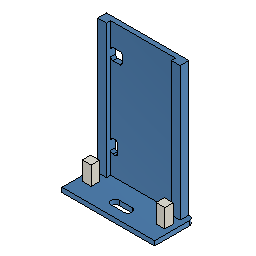
Base Station Enclosure Assembly (Autodesk Fusion 360 archive; units mm, degrees)
design "V2 enclosure Lid"
Autodesk Fusion 360 part; units mm, degrees
sketch "Sketch1" plane through (0, 0, 0) normal (0, 0, 1) x (1, 0, 0)
  line L0 (0, 0) -> (40, 0)
  line L1 (40, 0) -> (40, 17)
  line L2 (40, 17) -> (0, 17)
  line L3 (0, 17) -> (0, 0)
  line L4 (0, 0) -> (0, 6.6)
  line L5 (0, 0) -> (0, 2)
  line L6 (0, 2) -> (40, 2)
  line L7 (0, 17) -> (0, 15)
  line L8 (0, 15) -> (40, 15)
  line L9 (20, 0) -> (20, 4)
  line L10 (20, 4) -> (15.5, 4)
  line L11 (15.5, 4) -> (15.5, 7.5)
  line L12 (20, 4) -> (24.5, 4)
  line L13 (24.5, 4) -> (24.5, 7.5)
  line L14 (15.5, 7.5) -> (24.5, 7.5)
  line L15 (0, 6.6) -> (0, 10.2)
  line L16 (0, 10.2) -> (6, 10.2)
  line L17 (6, 10.2) -> (6, 6.6)
  line L18 (6, 6.6) -> (0, 6.6)
  line L19 (0, 17) -> (2.2, 17)
  line L20 (2.2, 17) -> (2.2, 0)
  line L21 (2.2, 15) -> (6, 15)
  line L22 (6, 15) -> (6, 13.2)
  line L23 (6, 13.2) -> (2.2, 13.2)
  line L24 (34, 6.6) -> (40, 6.6)
  line L25 (34, 10.2) -> (34, 6.6)
  line L26 (40, 10.2) -> (34, 10.2)
  line L27 (34, 13.2) -> (37.8, 13.2)
  line L28 (34, 15) -> (34, 13.2)
  line L29 (37.8, 17) -> (37.8, 0)
  dimension "d1" = 40
  dimension "d2" = 17
  dimension "d3" = 6.6
  dimension "d9" = 2
  dimension "d10" = 2
  dimension "d11" = 4
  dimension "d12" = 4.5
  dimension "d13" = 3.5
  dimension "d14" = 3.6
  dimension "d15" = 6
  dimension "d16" = 2.2
  dimension "d17" = 3.8
  dimension "d18" = 1.8
  constraint horizontal L0
  constraint vertical L1
  constraint horizontal L2
  constraint vertical L3
  constraint coincident L0.start L3.end
  constraint perpendicular L0 L4
  constraint perpendicular L0 L5
  constraint coincident L1 L6.end
  constraint perpendicular L1 L6
  constraint perpendicular L2 L7
  constraint coincident L1 L8.end
  constraint perpendicular L1 L8
  constraint midpoint L0 L9.start
  constraint perpendicular L6 L9
  constraint perpendicular L9 L10
  constraint perpendicular L6 L11
  constraint symmetric L10.start L9 L12.start
  constraint symmetric L9 L10.end L12.end
  constraint symmetric L9 L11.end L13.end
  constraint parallel L3 L15
  constraint perpendicular L3 L16
  constraint perpendicular L16 L17
  constraint perpendicular L4 L18
  constraint perpendicular L3 L19
  constraint coincident L0 L20.end
  constraint perpendicular L0 L20
  constraint coincident L8 L21.start
  constraint coincident L20 L21.start
  constraint perpendicular L20 L21
  constraint perpendicular L21 L22
  constraint coincident L20 L23.end
  constraint perpendicular L20 L23
  constraint symmetric L4.end L9 L24.end
  constraint symmetric L9 L15.end L26.start
  constraint symmetric L9 L16.end L25.start
  constraint symmetric L9 L17.end L24.start
  constraint symmetric L9 L19.end L29.start
  constraint symmetric L9 L20.end L29.end
  constraint symmetric L9 L21.end L28.start
  constraint symmetric L9 L22.end L27.start
  constraint symmetric L9 L23.end L27.end
  measures "d1" distance of L0.start L0.end
  measures "d2" distance of L0.start L2.end
  measures "d3" distance of L0.start L4.end
  measures "d9" distance of L0.start L5.end
  measures "d10" distance of L2.end L7.end
  measures "d11" distance of L9.start L9.end
  measures "d12" distance of L9.end L10.end
  measures "d13" distance of L10.end L11.end
  measures "d14" distance of L4.end L15.end
  measures "d15" distance of L15.end L16.end
  measures "d16" distance of L2.end L19.end
  measures "d17" distance of L21.start L21.end
  measures "d18" distance of L21.end L22.end
extrude "Extrude1" add sketch "Sketch1" along normal blind 2
extrude "Extrude2" add sketch "Sketch1" along normal blind 59.8 contours L2 L8 L20 L21 L29
fillet "Fillet1" [suppressed]
extrude "Extrude3" add sketch "Sketch1" along normal blind 59.8 contours L8 L20 L21 L22 L23 | L8 L27 L28 L29
extrude "Extrude4" add sketch "Sketch1" along normal blind 10 contours L16 L17 L18 L20 | L24 L25 L26 L29
fillet "Fillet2" radius 1.75 4 edges at (24.5, 7.5, 1) (24.5, 4, 1) (15.5, 4, 1) (15.5, 7.5, 1)
sketch "Sketch3" plane through (0, 17, 0) normal (0, 1, 0) x (-1, 0, 0)
  line L0 (0, 2) -> (-2.2, 2)
  line L1 (-2.2, 2) -> (-2.2, 59.8)
  line L2 (-2.2, 59.8) -> (-37.8, 59.8)
  line L3 (-37.8, 59.8) -> (-37.8, 2)
  line L4 (-40, 0) -> (0, 0)
  line L5 (0, 0) -> (0, 2)
  line L6 (-37.8, 2) -> (-40, 2)
  line L7 (-40, 2) -> (-40, 0)
  spline S0 degree 2 poles (-14.8194, 30.1777) (-15.2026, 30.1707) (-15.4828, 30.9322) knots 0 0 0 1 1 1
  spline S1 degree 2 poles (-15.4828, 30.9322) (-15.7629, 31.6937) (-15.7832, 32.8006) knots 0 0 0 1 1 1
  spline S2 degree 2 poles (-15.7832, 32.8006) (-15.8036, 33.9147) (-15.5287, 35.5737) knots 0 0 0 1 1 1
  spline S3 degree 2 poles (-15.5287, 35.5737) (-15.9989, 36.4382) (-16.9027, 37.1457) knots 0 0 0 1 1 1
  spline S4 degree 2 poles (-16.9027, 37.1457) (-17.8065, 37.8531) (-19.4538, 38.6535) knots 0 0 0 1 1 1
  spline S5 degree 2 poles (-19.4538, 38.6535) (-21.1011, 39.4538) (-21.651, 39.8306) knots 0 0 0 1 1 1
  spline S6 degree 2 poles (-21.651, 39.8306) (-22.201, 40.2074) (-22.7242, 40.8722) knots 0 0 0 1 1 1
  spline S7 degree 2 poles (-22.7242, 40.8722) (-24.0767, 42.6291) (-24.1118, 44.545) knots 0 0 0 1 1 1
  spline S8 degree 2 poles (-24.1118, 44.545) (-24.1305, 45.5669) (-23.7096, 46.2241) knots 0 0 0 1 1 1
  spline S9 degree 2 poles (-23.7096, 46.2241) (-23.2886, 46.8813) (-22.6003, 46.8939) knots 0 0 0 1 1 1
  spline S10 degree 2 poles (-22.6003, 46.8939) (-22.2526, 46.9003) (-22.0004, 46.699) knots 0 0 0 1 1 1
  spline S11 degree 2 poles (-22.0004, 46.699) (-21.7483, 46.4978) (-21.7431, 46.214) knots 0 0 0 1 1 1
  spline S12 degree 2 poles (-21.7431, 46.214) (-21.7347, 45.7527) (-22.2172, 45.7439) knots 0 0 0 1 1 1
  spline S13 degree 2 poles (-22.2172, 45.7439) (-22.4443, 45.7397) (-22.6101, 45.8787) knots 0 0 0 1 1 1
  spline S14 degree 2 poles (-22.6101, 45.8787) (-22.7759, 46.0176) (-22.7797, 46.2234) knots 0 0 0 1 1 1
  spline S15 degree 2 poles (-22.7797, 46.2234) (-22.7858, 46.5569) (-22.4594, 46.5629) knots 0 0 0 1 1 1
  spline S16 degree 2 poles (-22.4594, 46.5629) (-22.289, 46.566) (-22.2901, 46.6227) knots 0 0 0 1 1 1
  spline S17 degree 2 poles (-22.2901, 46.6227) (-22.2923, 46.7434) (-22.64, 46.737) knots 0 0 0 1 1 1
  spline S18 degree 2 poles (-22.64, 46.737) (-23.2148, 46.7265) (-23.6013, 46.1267) knots 0 0 0 1 1 1
  spline S19 degree 2 poles (-23.6013, 46.1267) (-23.9878, 45.5269) (-23.972, 44.6612) knots 0 0 0 1 1 1
  spline S20 degree 2 poles (-23.972, 44.6612) (-23.9371, 42.7594) (-22.1922, 41.2794) knots 0 0 0 1 1 1
  spline S21 degree 2 poles (-22.1922, 41.2794) (-21.3774, 40.5845) (-19.5118, 39.4971) knots 0 0 0 1 1 1
  spline S22 degree 2 poles (-19.5118, 39.4971) (-16.4838, 37.7212) (-15.5035, 35.7445) knots 0 0 0 1 1 1
  spline S23 degree 2 poles (-15.5035, 35.7445) (-15.4466, 36.1289) (-15.2904, 36.8984) knots 0 0 0 1 1 1
  spline S24 degree 2 poles (-15.2904, 36.8984) (-14.9331, 38.7079) (-14.9507, 39.6659) knots 0 0 0 1 1 1
  spline S25 degree 2 poles (-14.9507, 39.6659) (-14.9525, 39.7652) (-14.99, 40.2614) knots 0 0 0 1 1 1
  spline S26 degree 2 poles (-14.99, 40.2614) (-15.6083, 39.9165) (-16.4102, 39.9018) knots 0 0 0 1 1 1
  spline S27 degree 2 poles (-16.4102, 39.9018) (-17.9713, 39.8732) (-19.3625, 41.0331) knots 0 0 0 1 1 1
  spline S28 degree 2 poles (-19.3625, 41.0331) (-20.7538, 42.1931) (-20.7785, 43.5413) knots 0 0 0 1 1 1
  spline S29 degree 2 poles (-20.7785, 43.5413) (-20.7887, 44.1019) (-20.4226, 44.46) knots 0 0 0 1 1 1
  spline S30 degree 2 poles (-20.4226, 44.46) (-20.0565, 44.8181) (-19.4675, 44.8289) knots 0 0 0 1 1 1
  spline S31 degree 2 poles (-19.4675, 44.8289) (-18.6586, 44.8437) (-17.6646, 44.2479) knots 0 0 0 1 1 1
  spline S32 degree 2 poles (-17.6646, 44.2479) (-16.6705, 43.6521) (-15.9182, 42.6898) knots 0 0 0 1 1 1
  spline S33 degree 2 poles (-15.9182, 42.6898) (-15.1659, 41.7276) (-14.8536, 40.5691) knots 0 0 0 1 1 1
  spline S34 degree 2 poles (-14.8536, 40.5691) (-14.1046, 41.1432) (-14.1236, 42.1786) knots 0 0 0 1 1 1
  spline S35 degree 2 poles (-14.1236, 42.1786) (-14.1395, 43.0507) (-14.6641, 43.9313) knots 0 0 0 1 1 1
  spline S36 degree 2 poles (-14.6641, 43.9313) (-15.1887, 44.812) (-16.0755, 45.4696) knots 0 0 0 1 1 1
  spline S37 degree 2 poles (-16.0755, 45.4696) (-16.2122, 45.5664) (-16.2129, 45.6019) knots 0 0 0 1 1 1
  spline S38 degree 2 poles (-16.2129, 45.6019) (-16.2137, 45.6444) (-16.1713, 45.6594) knots 0 0 0 1 1 1
  spline S39 degree 2 poles (-16.1713, 45.6594) (-16.0505, 45.6616) (-15.457, 45.0908) knots 0 0 0 1 1 1
  spline S40 degree 2 poles (-15.457, 45.0908) (-14.0382, 43.7194) (-14.0103, 42.1947) knots 0 0 0 1 1 1
  spline S41 degree 2 poles (-14.0103, 42.1947) (-13.9886, 41.0105) (-14.8075, 40.3783) knots 0 0 0 1 1 1
  spline S42 degree 2 poles (-14.8075, 40.3783) (-14.5434, 39.5243) (-14.523, 38.4102) knots 0 0 0 1 1 1
  spline S43 degree 2 poles (-14.523, 38.4102) (-14.5125, 37.8354) (-14.5748, 37.3587) knots 0 0 0 1 1 1
  spline S44 degree 2 poles (-14.5748, 37.3587) (-14.6436, 36.8534) (-15.0121, 34.8804) knots 0 0 0 1 1 1
  spline S45 degree 2 poles (-15.0121, 34.8804) (-14.2653, 33.2543) (-14.2376, 31.7429) knots 0 0 0 1 1 1
  spline S46 degree 2 poles (-14.2376, 31.7429) (-14.2092, 30.1889) (-14.8194, 30.1777) knots 0 0 0 1 1 1
  spline S47 degree 2 poles (-14.8357, 30.291) (-14.6299, 30.2947) (-14.4953, 30.6983) knots 0 0 0 1 1 1
  spline S48 degree 2 poles (-14.4953, 30.6983) (-14.3608, 31.1018) (-14.372, 31.712) knots 0 0 0 1 1 1
  spline S49 degree 2 poles (-14.372, 31.712) (-14.3998, 33.2306) (-15.0645, 34.6452) knots 0 0 0 1 1 1
  spline S50 degree 2 poles (-15.0645, 34.6452) (-15.0897, 34.4673) (-15.2176, 33.6983) knots 0 0 0 1 1 1
  spline S51 degree 2 poles (-15.2176, 33.6983) (-15.4167, 32.5589) (-15.4006, 31.679) knots 0 0 0 1 1 1
  spline S52 degree 2 poles (-15.4006, 31.679) (-15.3901, 31.1042) (-15.2229, 30.6956) knots 0 0 0 1 1 1
  spline S53 degree 2 poles (-15.2229, 30.6956) (-15.0557, 30.2869) (-14.8357, 30.291) knots 0 0 0 1 1 1
  spline S54 degree 2 poles (-16.0675, 40.1849) (-15.4998, 40.1953) (-15.0221, 40.4667) knots 0 0 0 1 1 1
  spline S55 degree 2 poles (-15.0221, 40.4667) (-15.3138, 42.0514) (-16.7155, 43.3957) knots 0 0 0 1 1 1
  spline S56 degree 2 poles (-16.7155, 43.3957) (-18.1172, 44.74) (-19.4513, 44.7156) knots 0 0 0 1 1 1
  spline S57 degree 2 poles (-19.4513, 44.7156) (-19.9622, 44.7062) (-20.3041, 44.3841) knots 0 0 0 1 1 1
  spline S58 degree 2 poles (-20.3041, 44.3841) (-20.646, 44.0619) (-20.6376, 43.6007) knots 0 0 0 1 1 1
  spline S59 degree 2 poles (-20.6376, 43.6007) (-20.6156, 42.4015) (-19.115, 41.279) knots 0 0 0 1 1 1
  spline S60 degree 2 poles (-19.115, 41.279) (-17.6145, 40.1566) (-16.0675, 40.1849) knots 0 0 0 1 1 1
  spline S61 degree 2 poles (-21.3918, 34.5896) (-21.4131, 34.5892) (-21.5784, 34.7141) knots 0 0 0 1 1 1
  line L8 (-21.5784, 34.7141) -> (-21.9665, 35.0124)
  spline S62 degree 2 poles (-21.9665, 35.0124) (-23.8074, 36.4494) (-23.8266, 37.5005) knots 0 0 0 1 1 1
  spline S63 degree 2 poles (-23.8266, 37.5005) (-23.8357, 37.9977) (-23.4835, 38.3416) knots 0 0 0 1 1 1
  spline S64 degree 2 poles (-23.4835, 38.3416) (-23.1314, 38.6855) (-22.5921, 38.6954) knots 0 0 0 1 1 1
  spline S65 degree 2 poles (-22.5921, 38.6954) (-21.3148, 38.7188) (-20.31, 36.9555) knots 0 0 0 1 1 1
  spline S66 degree 2 poles (-20.31, 36.9555) (-19.7819, 36.0282) (-19.7711, 35.4392) knots 0 0 0 1 1 1
  spline S67 degree 2 poles (-19.7711, 35.4392) (-19.7665, 35.1837) (-19.9157, 35) knots 0 0 0 1 1 1
  spline S68 degree 2 poles (-19.9157, 35) (-20.065, 34.8162) (-20.2849, 34.8122) knots 0 0 0 1 1 1
  spline S69 degree 2 poles (-20.2849, 34.8122) (-20.7959, 34.8029) (-21.1664, 35.4633) knots 0 0 0 1 1 1
  spline S70 degree 2 poles (-21.1664, 35.4633) (-21.537, 36.1238) (-21.8778, 37.6792) knots 0 0 0 1 1 1
  spline S71 degree 2 poles (-21.8778, 37.6792) (-22.6175, 38.1483) (-23.1072, 38.1394) knots 0 0 0 1 1 1
  spline S72 degree 2 poles (-23.1072, 38.1394) (-23.7174, 38.1282) (-23.7053, 37.4676) knots 0 0 0 1 1 1
  spline S73 degree 2 poles (-23.7053, 37.4676) (-23.6848, 36.3453) (-21.4657, 34.7587) knots 0 0 0 1 1 1
  spline S74 degree 2 poles (-21.4657, 34.7587) (-21.3508, 34.6757) (-21.3497, 34.6188) knots 0 0 0 1 1 1
  spline S75 degree 2 poles (-21.3497, 34.6188) (-21.3563, 34.5903) (-21.3918, 34.5896) knots 0 0 0 1 1 1
  spline S76 degree 2 poles (-20.0864, 35.2134) (-19.8594, 35.2175) (-19.8639, 35.4659) knots 0 0 0 1 1 1
  spline S77 degree 2 poles (-19.8639, 35.4659) (-19.8708, 35.842) (-20.4036, 36.4462) knots 0 0 0 1 1 1
  spline S78 degree 2 poles (-20.4036, 36.4462) (-20.9364, 37.0505) (-21.7774, 37.6242) knots 0 0 0 1 1 1
  spline S79 degree 2 poles (-21.7774, 37.6242) (-21.4962, 36.6072) (-21.0042, 35.9064) knots 0 0 0 1 1 1
  spline S80 degree 2 poles (-21.0042, 35.9064) (-20.5122, 35.2056) (-20.0864, 35.2134) knots 0 0 0 1 1 1
  spline S81 degree 2 poles (-21.2933, 29.6012) (-21.4425, 29.5985) (-22.6909, 30.6131) knots 0 0 0 1 1 1
  spline S82 degree 2 poles (-22.6909, 30.6131) (-23.7155, 31.433) (-23.7243, 31.9161) knots 0 0 0 1 1 1
  spline S83 degree 2 poles (-23.7243, 31.9161) (-23.7303, 32.2429) (-23.4893, 32.4534) knots 0 0 0 1 1 1
  spline S84 degree 2 poles (-23.4893, 32.4534) (-23.2482, 32.6639) (-22.8792, 32.6707) knots 0 0 0 1 1 1
  spline S85 degree 2 poles (-22.8792, 32.6707) (-22.496, 32.6777) (-22.0448, 32.4588) knots 0 0 0 1 1 1
  spline S86 degree 2 poles (-22.0448, 32.4588) (-23.0513, 33.1502) (-23.4059, 33.5199) knots 0 0 0 1 1 1
  spline S87 degree 2 poles (-23.4059, 33.5199) (-23.7605, 33.8896) (-23.767, 34.2444) knots 0 0 0 1 1 1
  spline S88 degree 2 poles (-23.767, 34.2444) (-23.7739, 34.6205) (-23.4557, 34.8819) knots 0 0 0 1 1 1
  spline S89 degree 2 poles (-23.4557, 34.8819) (-23.1375, 35.1433) (-22.6478, 35.1522) knots 0 0 0 1 1 1
  spline S90 degree 2 poles (-22.6478, 35.1522) (-21.2854, 35.1772) (-20.2, 33.2734) knots 0 0 0 1 1 1
  spline S91 degree 2 poles (-20.2, 33.2734) (-19.7162, 32.4376) (-19.7067, 31.9195) knots 0 0 0 1 1 1
  spline S92 degree 2 poles (-19.7067, 31.9195) (-19.6986, 31.4796) (-20.1244, 31.4718) knots 0 0 0 1 1 1
  spline S93 degree 2 poles (-20.1244, 31.4718) (-20.245, 31.4696) (-20.4447, 31.5227) knots 0 0 0 1 1 1
  line L9 (-20.4447, 31.5227) -> (-19.7498, 31.1734)
  spline S94 degree 2 poles (-19.7498, 31.1734) (-19.7956, 30.9596) (-19.7926, 30.7964) knots 0 0 0 1 1 1
  spline S95 degree 2 poles (-19.7926, 30.7964) (-19.7891, 30.6048) (-19.7338, 30.3006) knots 0 0 0 1 1 1
  line L10 (-19.7338, 30.3006) -> (-21.8359, 31.5185)
  spline S96 degree 2 poles (-21.8359, 31.5185) (-22.9407, 32.1513) (-23.2884, 32.145) knots 0 0 0 1 1 1
  spline S97 degree 2 poles (-23.2884, 32.145) (-23.6219, 32.1389) (-23.6168, 31.8618) knots 0 0 0 1 1 1
  spline S98 degree 2 poles (-23.6168, 31.8618) (-23.6116, 31.5775) (-22.9499, 30.9641) knots 0 0 0 1 1 1
  spline S99 degree 2 poles (-22.9499, 30.9641) (-22.2882, 30.3506) (-21.3239, 29.7215) knots 0 0 0 1 1 1
  spline S100 degree 2 poles (-21.3239, 29.7215) (-21.2521, 29.6801) (-21.2515, 29.6446) knots 0 0 0 1 1 1
  spline S101 degree 2 poles (-21.2515, 29.6446) (-21.2507, 29.602) (-21.2933, 29.6012) knots 0 0 0 1 1 1
  spline S102 degree 2 poles (-20.1547, 31.5777) (-19.807, 31.5841) (-19.8128, 31.9034) knots 0 0 0 1 1 1
  spline S103 degree 2 poles (-19.8128, 31.9034) (-19.8248, 32.5562) (-21.1215, 33.5937) knots 0 0 0 1 1 1
  spline S104 degree 2 poles (-21.1215, 33.5937) (-22.4182, 34.6312) (-23.2059, 34.6167) knots 0 0 0 1 1 1
  spline S105 degree 2 poles (-23.2059, 34.6167) (-23.6672, 34.6083) (-23.6596, 34.1967) knots 0 0 0 1 1 1
  spline S106 degree 2 poles (-23.6596, 34.1967) (-23.6506, 33.7071) (-22.0036, 32.5305) knots 0 0 0 1 1 1
  spline S107 degree 2 poles (-22.0036, 32.5305) (-20.6514, 31.5686) (-20.1547, 31.5777) knots 0 0 0 1 1 1
  spline S108 degree 2 poles (-21.1485, 21.6963) (-21.1699, 21.703) (-21.2635, 21.7651) knots 0 0 0 1 1 1
  line L11 (-21.2635, 21.7651) -> (-21.6884, 22.0629)
  spline S109 degree 2 poles (-21.6884, 22.0629) (-23.5677, 23.3645) (-23.5794, 24.004) knots 0 0 0 1 1 1
  spline S110 degree 2 poles (-23.5794, 24.004) (-23.5855, 24.3379) (-23.341, 24.5556) knots 0 0 0 1 1 1
  spline S111 degree 2 poles (-23.341, 24.5556) (-23.0966, 24.7732) (-22.7063, 24.7804) knots 0 0 0 1 1 1
  spline S112 degree 2 poles (-22.7063, 24.7804) (-22.3089, 24.7877) (-21.8427, 24.5265) knots 0 0 0 1 1 1
  spline S113 degree 2 poles (-21.8427, 24.5265) (-21.7567, 24.4783) (-21.074, 24.0224) knots 0 0 0 1 1 1
  spline S114 degree 2 poles (-21.074, 24.0224) (-20.2115, 23.4419) (-19.949, 23.4467) knots 0 0 0 1 1 1
  spline S115 degree 2 poles (-19.949, 23.4467) (-19.658, 23.452) (-19.6634, 23.743) knots 0 0 0 1 1 1
  spline S116 degree 2 poles (-19.6634, 23.743) (-19.6805, 24.6796) (-23.5683, 26.887) knots 0 0 0 1 1 1
  spline S117 degree 2 poles (-23.5683, 26.887) (-23.5425, 27.0295) (-23.5471, 27.2778) knots 0 0 0 1 1 1
  spline S118 degree 2 poles (-23.5471, 27.2778) (-23.5524, 27.5688) (-23.5846, 27.774) knots 0 0 0 1 1 1
  line L12 (-23.5846, 27.774) -> (-21.9695, 26.7956)
  spline S119 degree 2 poles (-21.9695, 26.7956) (-20.3761, 25.8381) (-20.0213, 25.8446) knots 0 0 0 1 1 1
  spline S120 degree 2 poles (-20.0213, 25.8446) (-19.702, 25.8505) (-19.7068, 26.113) knots 0 0 0 1 1 1
  spline S121 degree 2 poles (-19.7068, 26.113) (-19.7139, 26.5033) (-20.8514, 27.3698) knots 0 0 0 1 1 1
  spline S122 degree 2 poles (-20.8514, 27.3698) (-21.9888, 28.2363) (-23.6085, 29.0797) knots 0 0 0 1 1 1
  spline S123 degree 2 poles (-23.6085, 29.0797) (-23.5831, 29.2434) (-23.5878, 29.4989) knots 0 0 0 1 1 1
  spline S124 degree 2 poles (-23.5878, 29.4989) (-23.5928, 29.7756) (-23.625, 29.9809) knots 0 0 0 1 1 1
  line L13 (-23.625, 29.9809) -> (-22.0098, 28.9954)
  spline S125 degree 2 poles (-22.0098, 28.9954) (-20.3443, 27.9753) (-19.954, 27.9825) knots 0 0 0 1 1 1
  spline S126 degree 2 poles (-19.954, 27.9825) (-19.7411, 27.9864) (-19.7441, 28.1499) knots 0 0 0 1 1 1
  spline S127 degree 2 poles (-19.7441, 28.1499) (-19.7505, 28.4984) (-21.2927, 29.5655) knots 0 0 0 1 1 1
  spline S128 degree 2 poles (-21.2927, 29.5655) (-21.3933, 29.6348) (-21.3941, 29.6775) knots 0 0 0 1 1 1
  spline S129 degree 2 poles (-21.3941, 29.6775) (-21.3875, 29.706) (-21.352, 29.7066) knots 0 0 0 1 1 1
  spline S130 degree 2 poles (-21.352, 29.7066) (-21.2883, 29.7078) (-20.4549, 29.069) knots 0 0 0 1 1 1
  spline S131 degree 2 poles (-20.4549, 29.069) (-19.643, 28.4439) (-19.6366, 28.0957) knots 0 0 0 1 1 1
  spline S132 degree 2 poles (-19.6366, 28.0957) (-19.6325, 27.8683) (-19.8459, 27.7008) knots 0 0 0 1 1 1
  spline S133 degree 2 poles (-19.8459, 27.7008) (-20.0593, 27.5334) (-20.3574, 27.5279) knots 0 0 0 1 1 1
  spline S134 degree 2 poles (-20.3574, 27.5279) (-20.7689, 27.5204) (-21.5075, 27.9256) knots 0 0 0 1 1 1
  spline S135 degree 2 poles (-21.5075, 27.9256) (-19.6107, 26.6827) (-19.5993, 26.0582) knots 0 0 0 1 1 1
  spline S136 degree 2 poles (-19.5993, 26.0582) (-19.5938, 25.7602) (-19.8316, 25.5642) knots 0 0 0 1 1 1
  spline S137 degree 2 poles (-19.8316, 25.5642) (-20.0694, 25.3682) (-20.4313, 25.3615) knots 0 0 0 1 1 1
  spline S138 degree 2 poles (-20.4313, 25.3615) (-20.8357, 25.3541) (-21.4671, 25.7188) knots 0 0 0 1 1 1
  spline S139 degree 2 poles (-21.4671, 25.7188) (-19.569, 24.4048) (-19.5567, 23.7307) knots 0 0 0 1 1 1
  spline S140 degree 2 poles (-19.5567, 23.7307) (-19.5511, 23.4256) (-19.8098, 23.2114) knots 0 0 0 1 1 1
  spline S141 degree 2 poles (-19.8098, 23.2114) (-20.0685, 22.9973) (-20.4446, 22.9904) knots 0 0 0 1 1 1
  spline S142 degree 2 poles (-20.4446, 22.9904) (-20.8846, 22.9824) (-21.4799, 23.3193) knots 0 0 0 1 1 1
  spline S143 degree 2 poles (-21.4799, 23.3193) (-21.4871, 23.3262) (-22.3994, 23.9129) knots 0 0 0 1 1 1
  spline S144 degree 2 poles (-22.3994, 23.9129) (-22.9167, 24.2512) (-23.1863, 24.2463) knots 0 0 0 1 1 1
  spline S145 degree 2 poles (-23.1863, 24.2463) (-23.4772, 24.241) (-23.4719, 23.9496) knots 0 0 0 1 1 1
  spline S146 degree 2 poles (-23.4719, 23.9496) (-23.4618, 23.3953) (-21.6473, 22.1491) knots 0 0 0 1 1 1
  line L14 (-21.6473, 22.1491) -> (-21.3377, 21.9345)
  line L15 (-21.3377, 21.9345) -> (-21.179, 21.8094)
  spline S147 degree 2 poles (-21.179, 21.8094) (-21.1073, 21.7751) (-21.1067, 21.7396) knots 0 0 0 1 1 1
  spline S148 degree 2 poles (-21.1067, 21.7396) (-21.1059, 21.697) (-21.1485, 21.6963) knots 0 0 0 1 1 1
  spline S149 degree 2 poles (-17.6126, 13.8995) (-19.2386, 13.8697) (-21.1073, 15.4599) knots 0 0 0 1 1 1
  spline S150 degree 2 poles (-21.1073, 15.4599) (-23.3803, 17.3974) (-23.4111, 19.0781) knots 0 0 0 1 1 1
  spline S151 degree 2 poles (-23.4111, 19.0781) (-23.4267, 19.9312) (-22.8289, 20.4861) knots 0 0 0 1 1 1
  spline S152 degree 2 poles (-22.8289, 20.4861) (-22.2312, 21.0411) (-21.2788, 21.0586) knots 0 0 0 1 1 1
  spline S153 degree 2 poles (-21.2788, 21.0586) (-19.3712, 21.0935) (-17.3568, 18.7865) knots 0 0 0 1 1 1
  spline S154 degree 2 poles (-17.3568, 18.7865) (-15.6248, 16.7938) (-15.6027, 15.5867) knots 0 0 0 1 1 1
  spline S155 degree 2 poles (-15.6027, 15.5867) (-15.589, 14.8362) (-16.1403, 14.3763) knots 0 0 0 1 1 1
  spline S156 degree 2 poles (-16.1403, 14.3763) (-16.6917, 13.9164) (-17.6126, 13.8995) knots 0 0 0 1 1 1
  spline S157 degree 2 poles (-16.8415, 14.4318) (-15.6813, 14.4531) (-15.7018, 15.5707) knots 0 0 0 1 1 1
  spline S158 degree 2 poles (-15.7018, 15.5707) (-15.7186, 16.4868) (-16.8185, 17.6671) knots 0 0 0 1 1 1
  spline S159 degree 2 poles (-16.8185, 17.6671) (-17.8607, 18.7917) (-19.3154, 19.5819) knots 0 0 0 1 1 1
  spline S160 degree 2 poles (-19.3154, 19.5819) (-20.8416, 20.4064) (-21.9976, 20.3852) knots 0 0 0 1 1 1
  spline S161 degree 2 poles (-21.9976, 20.3852) (-23.3352, 20.3607) (-23.312, 19.0941) knots 0 0 0 1 1 1
  spline S162 degree 2 poles (-23.312, 19.0941) (-23.2834, 17.5341) (-21.0749, 15.9999) knots 0 0 0 1 1 1
  spline S163 degree 2 poles (-21.0749, 15.9999) (-20.0317, 15.2742) (-18.8733, 14.845) knots 0 0 0 1 1 1
  spline S164 degree 2 poles (-18.8733, 14.845) (-17.7148, 14.4158) (-16.8415, 14.4318) knots 0 0 0 1 1 1
  spline S165 degree 2 poles (-16.7428, 7.3707) (-18.4229, 7.3399) (-18.9868, 10.2542) knots 0 0 0 1 1 1
  spline S166 degree 2 poles (-18.9868, 10.2542) (-19.346, 8.5298) (-20.7024, 8.5049) knots 0 0 0 1 1 1
  spline S167 degree 2 poles (-20.7024, 8.5049) (-21.7252, 8.4862) (-22.5207, 9.6418) knots 0 0 0 1 1 1
  spline S168 degree 2 poles (-22.5207, 9.6418) (-23.3162, 10.7974) (-23.3443, 12.3358) knots 0 0 0 1 1 1
  spline S169 degree 2 poles (-23.3443, 12.3358) (-23.3622, 13.3095) (-22.9834, 13.9421) knots 0 0 0 1 1 1
  spline S170 degree 2 poles (-22.9834, 13.9421) (-22.6045, 14.5747) (-21.9943, 14.5859) knots 0 0 0 1 1 1
  spline S171 degree 2 poles (-21.9943, 14.5859) (-21.3627, 14.5975) (-20.9043, 13.9847) knots 0 0 0 1 1 1
  spline S172 degree 2 poles (-20.9043, 13.9847) (-20.4459, 13.372) (-20.4298, 12.4921) knots 0 0 0 1 1 1
  spline S173 degree 2 poles (-20.4298, 12.4921) (-20.4175, 11.8251) (-20.5027, 11.8235) knots 0 0 0 1 1 1
  spline S174 degree 2 poles (-20.5027, 11.8235) (-20.5453, 11.8228) (-20.546, 11.8653) knots 0 0 0 1 1 1
  line L16 (-20.546, 11.8653) -> (-20.5471, 11.9221)
  spline S175 degree 2 poles (-20.5471, 11.9221) (-20.5093, 12.1854) (-20.5126, 12.3628) knots 0 0 0 1 1 1
  spline S176 degree 2 poles (-20.5126, 12.3628) (-20.5267, 13.1363) (-20.9801, 13.6639) knots 0 0 0 1 1 1
  spline S177 degree 2 poles (-20.9801, 13.6639) (-21.4334, 14.1916) (-22.072, 14.1799) knots 0 0 0 1 1 1
  spline S178 degree 2 poles (-22.072, 14.1799) (-22.5971, 14.1702) (-22.9229, 13.7409) knots 0 0 0 1 1 1
  spline S179 degree 2 poles (-22.9229, 13.7409) (-23.2486, 13.3116) (-23.2364, 12.643) knots 0 0 0 1 1 1
  spline S180 degree 2 poles (-23.2364, 12.643) (-23.2126, 11.3458) (-22.2694, 10.2745) knots 0 0 0 1 1 1
  spline S181 degree 2 poles (-22.2694, 10.2745) (-21.3261, 9.2033) (-20.2183, 9.2236) knots 0 0 0 1 1 1
  spline S182 degree 2 poles (-20.2183, 9.2236) (-19.3021, 9.2404) (-19.0315, 10.3669) knots 0 0 0 1 1 1
  spline S183 degree 2 poles (-19.0315, 10.3669) (-19.1349, 10.9755) (-19.1421, 11.3658) knots 0 0 0 1 1 1
  spline S184 degree 2 poles (-19.1421, 11.3658) (-19.1488, 11.7348) (-19.0566, 11.7364) knots 0 0 0 1 1 1
  spline S185 degree 2 poles (-19.0566, 11.7364) (-18.9146, 11.739) (-18.905, 11.2139) knots 0 0 0 1 1 1
  spline S186 degree 2 poles (-18.905, 11.2139) (-18.8976, 10.8095) (-18.9605, 10.3682) knots 0 0 0 1 1 1
  spline S187 degree 2 poles (-18.9605, 10.3682) (-18.5792, 9.2962) (-17.887, 8.6701) knots 0 0 0 1 1 1
  spline S188 degree 2 poles (-17.887, 8.6701) (-17.1948, 8.0439) (-16.3937, 8.0585) knots 0 0 0 1 1 1
  spline S189 degree 2 poles (-16.3937, 8.0585) (-15.4935, 8.075) (-15.5146, 9.2246) knots 0 0 0 1 1 1
  spline S190 degree 2 poles (-15.5146, 9.2246) (-15.5328, 10.218) (-16.234, 11.199) knots 0 0 0 1 1 1
  spline S191 degree 2 poles (-16.234, 11.199) (-16.9352, 12.1799) (-17.6287, 12.1672) knots 0 0 0 1 1 1
  spline S192 degree 2 poles (-17.6287, 12.1672) (-18.2657, 12.1555) (-18.2507, 11.3359) knots 0 0 0 1 1 1
  spline S193 degree 2 poles (-18.2507, 11.3359) (-18.2417, 10.8471) (-17.8386, 10.2379) knots 0 0 0 1 1 1
  spline S194 degree 2 poles (-17.8386, 10.2379) (-17.4355, 9.6287) (-16.8924, 9.2844) knots 0 0 0 1 1 1
  spline S195 degree 2 poles (-16.8924, 9.2844) (-16.8212, 9.2502) (-16.8203, 9.2007) knots 0 0 0 1 1 1
  spline S196 degree 2 poles (-16.8203, 9.2007) (-16.8268, 9.1722) (-16.848, 9.1718) knots 0 0 0 1 1 1
  spline S197 degree 2 poles (-16.848, 9.1718) (-16.9256, 9.1704) (-17.2272, 9.4341) knots 0 0 0 1 1 1
  spline S198 degree 2 poles (-17.2272, 9.4341) (-17.5288, 9.6979) (-17.7167, 9.9284) knots 0 0 0 1 1 1
  spline S199 degree 2 poles (-17.7167, 9.9284) (-18.3236, 10.6685) (-18.3363, 11.3628) knots 0 0 0 1 1 1
  spline S200 degree 2 poles (-18.3363, 11.3628) (-18.344, 11.783) (-18.1047, 12.051) knots 0 0 0 1 1 1
  spline S201 degree 2 poles (-18.1047, 12.051) (-17.8653, 12.319) (-17.483, 12.326) knots 0 0 0 1 1 1
  spline S202 degree 2 poles (-17.483, 12.326) (-16.7681, 12.3391) (-16.109, 11.3432) knots 0 0 0 1 1 1
  spline S203 degree 2 poles (-16.109, 11.3432) (-15.45, 10.3473) (-15.4292, 9.212) knots 0 0 0 1 1 1
  spline S204 degree 2 poles (-15.4292, 9.212) (-15.414, 8.3817) (-15.77, 7.8819) knots 0 0 0 1 1 1
  spline S205 degree 2 poles (-15.77, 7.8819) (-16.126, 7.382) (-16.7428, 7.3707) knots 0 0 0 1 1 1
sketch "Sketch4" plane through (0, 17, 0) normal (0, 1, 0) x (-1, 0, 0)
  line L0 (-40, 0) -> (0, 0)
  line L1 (0, 0) -> (0, 2)
  line L2 (0, 2) -> (-2.2, 2)
  line L3 (-2.2, 2) -> (-2.2, 59.8)
  line L4 (-2.2, 59.8) -> (-37.8, 59.8)
  line L5 (-37.8, 59.8) -> (-37.8, 2)
  line L6 (-37.8, 2) -> (-40, 2)
  line L7 (-40, 2) -> (-40, 0)
  line L8 (-35.4636, 42.0484) -> (-35.4636, 17.9538) construction
  line L9 (-35.4636, 17.9538) -> (-7.8615, 17.9538) construction
  line L10 (-7.8615, 17.9538) -> (-7.8615, 42.0484) construction
  line L11 (-7.8615, 42.0484) -> (-35.4636, 42.0484) construction
  dimension "d45" = 6
  text T0 "TEAM\n03" font "Arial Black" height 6 align centre middle in box 24.0946 x 27.6021 at (-35.4636, 42.0484) x (0, -1) y (1, 0) spacing 1 kerned
extrude "Extrude8" cut sketch "Sketch4" against normal blind 1 text T0
sketch "Sketch5" plane through (0, 17, 0) normal (0, 1, 0) x (-1, 0, 0)
  line L0 (-18.7526, 31.3599) -> (-18.7526, 36.4185)
  line L1 (-18.7526, 36.4185) -> (-12.7526, 36.4185)
  line L2 (-12.7526, 36.4185) -> (-12.7526, 31.4499)
  line L3 (-12.7526, 31.4499) -> (-14.0336, 31.4499)
  line L4 (-14.0336, 31.4499) -> (-14.0336, 34.5604)
  line L5 (-14.0336, 34.5604) -> (-14.9873, 34.5604)
  line L6 (-14.9873, 34.5604) -> (-14.9873, 31.675)
  line L7 (-14.9873, 31.675) -> (-16.211, 31.675)
  line L8 (-16.211, 31.675) -> (-16.211, 34.5604)
  line L9 (-16.211, 34.5604) -> (-17.3938, 34.5604)
  line L10 (-17.3938, 34.5604) -> (-17.3938, 31.3599)
  line L11 (-17.3938, 31.3599) -> (-18.7526, 31.3599)
  spline S0 degree 3 poles (-25.5057, 27.1239) (-25.5119, 27.2162) (-25.5238, 27.3939) (-25.6318, 27.5349) (-25.6837, 27.6027) knots 0 0 0 0 0.027074 0.052111 0.052111 0.052111 0.052111
  spline S1 degree 3 poles (-25.6837, 27.6027) (-25.7629, 27.6602) (-25.9488, 27.7952) (-26.1769, 27.8315) (-26.3079, 27.8524) knots 0 0 0 0 0.028969 0.068055 0.068055 0.068055 0.068055
  line L12 (-26.3079, 27.8524) -> (-26.0255, 29.4281)
  spline S2 degree 3 poles (-26.0255, 29.4281) (-25.7916, 29.3509) (-25.339, 29.2014) (-25.0237, 28.8451) (-24.8713, 28.673) knots 0 0 0 0 0.072436 0.140136 0.140136 0.140136 0.140136
  spline S3 degree 3 poles (-24.8713, 28.673) (-24.7547, 28.4525) (-24.4939, 27.9596) (-24.4786, 27.4003) (-24.4702, 27.0911) knots 0 0 0 0 0.073881 0.16514 0.16514 0.16514 0.16514
  spline S4 degree 3 poles (-24.4702, 27.0911) (-24.4753, 26.7449) (-24.4841, 26.1397) (-24.7811, 25.6165) (-24.9081, 25.3926) knots 0 0 0 0 0.101784 0.177892 0.177892 0.177892 0.177892
  spline S5 degree 3 poles (-24.9081, 25.3926) (-25.0625, 25.2398) (-25.3687, 24.9368) (-25.7969, 24.8913) (-26.0091, 24.8688) knots 0 0 0 0 0.063135 0.125208 0.125208 0.125208 0.125208
  spline S6 degree 3 poles (-26.0091, 24.8688) (-26.1353, 24.8774) (-26.3863, 24.8946) (-26.6046, 25.0195) (-26.713, 25.0816) knots 0 0 0 0 0.03742 0.074398 0.074398 0.074398 0.074398
  spline S7 degree 3 poles (-26.713, 25.0816) (-26.8171, 25.1658) (-27.04, 25.3461) (-27.1871, 25.5927) (-27.2656, 25.7241) knots 0 0 0 0 0.039844 0.085338 0.085338 0.085338 0.085338
  spline S8 degree 3 poles (-27.2656, 25.7241) (-27.2924, 25.6202) (-27.34, 25.4354) (-27.4278, 25.2661) (-27.4661, 25.1921) knots 0 0 0 0 0.032077 0.05702 0.05702 0.05702 0.05702
  spline S9 degree 3 poles (-27.4661, 25.1921) (-27.5321, 25.0982) (-27.6633, 24.9115) (-27.8555, 24.7886) (-27.9511, 24.7276) knots 0 0 0 0 0.034061 0.067736 0.067736 0.067736 0.067736
  spline S10 degree 3 poles (-27.9511, 24.7276) (-28.0595, 24.6792) (-28.2878, 24.5774) (-28.538, 24.5672) (-28.6694, 24.5618) knots 0 0 0 0 0.035262 0.074313 0.074313 0.074313 0.074313
  spline S11 degree 3 poles (-28.6694, 24.5618) (-28.8434, 24.5739) (-29.1964, 24.5984) (-29.5134, 24.756) (-29.6742, 24.836) knots 0 0 0 0 0.051769 0.105062 0.105062 0.105062 0.105062
  spline S12 degree 3 poles (-29.6742, 24.836) (-29.8257, 24.9384) (-30.1323, 25.1456) (-30.32, 25.4646) (-30.415, 25.6259) knots 0 0 0 0 0.054141 0.109515 0.109515 0.109515 0.109515
  spline S13 degree 3 poles (-30.415, 25.6259) (-30.4906, 25.8226) (-30.6579, 26.2577) (-30.6688, 26.7247) (-30.6749, 26.9806) knots 0 0 0 0 0.062756 0.138852 0.138852 0.138852 0.138852
  spline S14 degree 3 poles (-30.6749, 26.9806) (-30.6714, 27.2267) (-30.6653, 27.6664) (-30.5384, 28.0868) (-30.4825, 28.2719) knots 0 0 0 0 0.073367 0.131116 0.131116 0.131116 0.131116
  spline S15 degree 3 poles (-30.4825, 28.2719) (-30.412, 28.4216) (-30.2732, 28.7163) (-30.0363, 28.9397) (-29.9197, 29.0495) knots 0 0 0 0 0.049159 0.096753 0.096753 0.096753 0.096753
  spline S16 degree 3 poles (-29.9197, 29.0495) (-29.784, 29.1465) (-29.4982, 29.3508) (-29.1641, 29.4605) (-28.9886, 29.5181) knots 0 0 0 0 0.049739 0.104776 0.104776 0.104776 0.104776
  line L13 (-28.9886, 29.5181) -> (-28.7676, 27.8524)
  spline S17 degree 3 poles (-28.7676, 27.8524) (-28.915, 27.8221) (-29.1705, 27.7696) (-29.3778, 27.6135) (-29.4654, 27.5475) knots 0 0 0 0 0.044421 0.076985 0.076985 0.076985 0.076985
  spline S18 degree 3 poles (-29.4654, 27.5475) (-29.5221, 27.4722) (-29.6393, 27.3167) (-29.6529, 27.1221) (-29.6598, 27.0215) knots 0 0 0 0 0.027641 0.057153 0.057153 0.057153 0.057153
  spline S19 degree 3 poles (-29.6598, 27.0215) (-29.6497, 26.9145) (-29.6296, 26.7011) (-29.4859, 26.5421) (-29.4143, 26.4629) knots 0 0 0 0 0.031354 0.062502 0.062502 0.062502 0.062502
  spline S20 degree 3 poles (-29.4143, 26.4629) (-29.322, 26.3979) (-29.1262, 26.2599) (-28.8863, 26.2468) (-28.7594, 26.2398) knots 0 0 0 0 0.033176 0.070431 0.070431 0.070431 0.070431
  spline S21 degree 3 poles (-28.7594, 26.2398) (-28.6317, 26.2456) (-28.3949, 26.2563) (-28.2018, 26.3921) (-28.1128, 26.4547) knots 0 0 0 0 0.037427 0.06941 0.06941 0.06941 0.06941
  spline S22 degree 3 poles (-28.1128, 26.4547) (-28.046, 26.5353) (-27.906, 26.704) (-27.8913, 26.9233) (-27.8836, 27.0379) knots 0 0 0 0 0.030607 0.064099 0.064099 0.064099 0.064099
  spline S23 degree 3 poles (-27.8836, 27.0379) (-27.8896, 27.1161) (-27.9038, 27.2993) (-27.9534, 27.4765) (-27.9818, 27.5782) knots 0 0 0 0 0.023458 0.055025 0.055025 0.055025 0.055025
  line L14 (-27.9818, 27.5782) -> (-26.7908, 27.4922)
  spline S24 degree 3 poles (-26.7908, 27.4922) (-26.7967, 27.451) (-26.8071, 27.379) (-26.81, 27.3064) (-26.8113, 27.2753) knots 0 0 0 0 0.012475 0.021801 0.021801 0.021801 0.021801
  spline S25 degree 3 poles (-26.8113, 27.2753) (-26.8034, 27.1715) (-26.7879, 26.9685) (-26.6634, 26.8076) (-26.6025, 26.7289) knots 0 0 0 0 0.030481 0.059646 0.059646 0.059646 0.059646
  spline S26 degree 3 poles (-26.6025, 26.7289) (-26.5305, 26.6651) (-26.3885, 26.5393) (-26.2001, 26.5196) (-26.1073, 26.51) knots 0 0 0 0 0.028112 0.055373 0.055373 0.055373 0.055373
  spline S27 degree 3 poles (-26.1073, 26.51) (-26.022, 26.5154) (-25.859, 26.5258) (-25.7306, 26.6259) (-25.6694, 26.6737) knots 0 0 0 0 0.024996 0.047731 0.047731 0.047731 0.047731
  spline S28 degree 3 poles (-25.6694, 26.6737) (-25.6217, 26.7359) (-25.5202, 26.8683) (-25.5107, 27.0354) (-25.5057, 27.1239) knots 0 0 0 0 0.022993 0.048899 0.048899 0.048899 0.048899
  spline S29 degree 3 poles (-29.7253, 34.6014) (-29.5967, 34.6712) (-29.3108, 34.8265) (-28.9934, 34.8991) (-28.8188, 34.939) knots 0 0 0 0 0.043723 0.097138 0.097138 0.097138 0.097138
  spline S30 degree 3 poles (-28.8188, 34.939) (-28.6175, 34.9742) (-28.1972, 35.0477) (-27.7704, 35.0556) (-27.548, 35.0597) knots 0 0 0 0 0.061196 0.127823 0.127823 0.127823 0.127823
  spline S31 degree 3 poles (-27.548, 35.0597) (-27.0496, 35.0561) (-26.194, 35.0497) (-25.4601, 34.6222) (-25.1537, 34.4438) knots 0 0 0 0 0.146209 0.250976 0.250976 0.250976 0.250976
  spline S32 degree 3 poles (-25.1537, 34.4438) (-24.9548, 34.1956) (-24.5181, 33.6508) (-24.4871, 32.9492) (-24.4702, 32.5673) knots 0 0 0 0 0.093096 0.204358 0.204358 0.204358 0.204358
  spline S33 degree 3 poles (-24.4702, 32.5673) (-24.4737, 32.382) (-24.4801, 32.0436) (-24.5761, 31.7194) (-24.6196, 31.5727) knots 0 0 0 0 0.055276 0.100975 0.100975 0.100975 0.100975
  spline S34 degree 3 poles (-24.6196, 31.5727) (-24.671, 31.4514) (-24.7688, 31.2202) (-24.9312, 31.0291) (-25.0084, 30.9383) knots 0 0 0 0 0.039263 0.074791 0.074791 0.074791 0.074791
  spline S35 degree 3 poles (-25.0084, 30.9383) (-25.0876, 30.8617) (-25.2407, 30.7136) (-25.4236, 30.6043) (-25.5118, 30.5516) knots 0 0 0 0 0.032935 0.063671 0.063671 0.063671 0.063671
  spline S36 degree 3 poles (-25.5118, 30.5516) (-25.6061, 30.5062) (-25.8041, 30.4108) (-26.0165, 30.3541) (-26.1278, 30.3244) knots 0 0 0 0 0.031307 0.06578 0.06578 0.06578 0.06578
  spline S37 degree 3 poles (-26.1278, 30.3244) (-26.3555, 30.2755) (-26.8168, 30.1763) (-27.2886, 30.1632) (-27.5275, 30.1566) knots 0 0 0 0 0.0697 0.141241 0.141241 0.141241 0.141241
  spline S38 degree 3 poles (-27.5275, 30.1566) (-28.009, 30.1629) (-28.8499, 30.1737) (-29.598, 30.5488) (-29.9177, 30.7091) knots 0 0 0 0 0.142078 0.248123 0.248123 0.248123 0.248123
  spline S39 degree 3 poles (-29.9177, 30.7091) (-30.1379, 30.9466) (-30.6307, 31.4779) (-30.6591, 32.2083) (-30.6749, 32.6123) knots 0 0 0 0 0.094237 0.210892 0.210892 0.210892 0.210892
  spline S40 degree 3 poles (-30.6749, 32.6123) (-30.6692, 32.8435) (-30.6588, 33.266) (-30.5036, 33.6583) (-30.4334, 33.836) knots 0 0 0 0 0.068717 0.1256 0.1256 0.1256 0.1256
  spline S41 degree 3 poles (-30.4334, 33.836) (-30.3424, 33.9852) (-30.158, 34.2879) (-29.8709, 34.4959) (-29.7253, 34.6014) knots 0 0 0 0 0.051861 0.105194 0.105194 0.105194 0.105194
  line L15 (-18.7526, 22.3435) -> (-18.7526, 23.8619)
  line L16 (-18.7526, 23.8619) -> (-12.7526, 23.8619)
  line L17 (-12.7526, 23.8619) -> (-12.7526, 21.4237)
  line L18 (-12.7526, 21.4237) -> (-16.4034, 20.4834)
  line L19 (-16.4034, 20.4834) -> (-12.7526, 19.5498)
  line L20 (-12.7526, 19.5498) -> (-12.7526, 17.113)
  line L21 (-12.7526, 17.113) -> (-18.7526, 17.113)
  line L22 (-18.7526, 17.113) -> (-18.7526, 18.6314)
  line L23 (-18.7526, 18.6314) -> (-14.1769, 18.6314)
  line L24 (-14.1769, 18.6314) -> (-18.7526, 19.8013)
  line L25 (-18.7526, 19.8013) -> (-18.7526, 21.1757)
  line L26 (-18.7526, 21.1757) -> (-14.1769, 22.3435)
  line L27 (-14.1769, 22.3435) -> (-18.7526, 22.3435)
  line L28 (-18.7526, 24.4308) -> (-18.7526, 26.3723)
  line L29 (-18.7526, 26.3723) -> (-17.7622, 26.6725)
  line L30 (-17.7622, 26.6725) -> (-17.7622, 28.7774)
  line L31 (-17.7622, 28.7774) -> (-18.7526, 29.0699)
  line L32 (-18.7526, 29.0699) -> (-18.7526, 30.9629)
  line L33 (-18.7526, 30.9629) -> (-12.7526, 28.7078)
  line L34 (-12.7526, 28.7078) -> (-12.7526, 26.6854)
  line L35 (-12.7526, 26.6854) -> (-18.7526, 24.4308)
  line L36 (-14.2342, 40.9984) -> (-14.2342, 42.8892)
  line L37 (-14.2342, 42.8892) -> (-12.7526, 42.8892)
  line L38 (-12.7526, 42.8892) -> (-12.7526, 37.2535)
  line L39 (-12.7526, 37.2535) -> (-14.2342, 37.2535)
  line L40 (-14.2342, 37.2535) -> (-14.2342, 39.1443)
  line L41 (-14.2342, 39.1443) -> (-18.7526, 39.1443)
  line L42 (-18.7526, 39.1443) -> (-18.7526, 40.9984)
  line L43 (-18.7526, 40.9984) -> (-14.2342, 40.9984)
  line L44 (-40, 0) -> (0, 0)
  line L45 (0, 0) -> (0, 2)
  line L46 (0, 2) -> (-2.2, 2)
  line L47 (-2.2, 2) -> (-2.2, 59.8)
  line L48 (-2.2, 59.8) -> (-37.8, 59.8)
  line L49 (-37.8, 59.8) -> (-37.8, 2)
  line L50 (-37.8, 2) -> (-40, 2)
  line L51 (-40, 2) -> (-40, 0)
  line L52 (-2.2, 59.8) -> (-6, 59.8)
  line L53 (-6, 59.8) -> (-6, 0)
  line L54 (-6, 50.2912) -> (-11, 50.2912)
  line L55 (-11, 50.2912) -> (-11, 45.2912)
  line L56 (-11, 45.2912) -> (-6, 45.2912)
  line L57 (-6, 45.2912) -> (-6, 50.2912)
  line L58 (-6, 10.3209) -> (-9, 10.3209)
  line L59 (-9, 10.3209) -> (-9, 16.3209)
  line L60 (-9, 16.3209) -> (-6, 16.3209)
  line L61 (-6, 16.3209) -> (-6, 10.3209)
  dimension "d48" = 3.8
  dimension "d49" = 5
  dimension "d50" = 5
  dimension "d51" = 3
  dimension "d52" = 6
  constraint coincident L47.end L48.start
  constraint perpendicular L47 L52
  constraint coincident L44 L53.end
  constraint perpendicular L44 L53
  constraint horizontal L54
  constraint vertical L55
  constraint horizontal L56
  constraint vertical L57
  constraint coincident L53 L54.start
  constraint horizontal L58
  constraint vertical L59
  constraint horizontal L60
  constraint vertical L61
  constraint coincident L53 L58.start
  measures "d48" distance of L47.end L52.end
  measures "d49" distance of L54.start L54.end
  measures "d50" distance of L54.start L56.end
  measures "d51" distance of L58.start L58.end
  measures "d52" distance of L58.start L60.end
extrude "Extrude9" cut sketch "Sketch5" against normal blind 14 contours L53 L58 L59 L60 L61 | L53 L54 L55 L56 L57
fillet "Fillet3" radius 1 8 edges at (11, 16, 45.2912) (6, 16, 45.2912) (6, 16, 50.2912) (11, 16, 50.2912) (6, 16, 10.3209) (6, 16, 16.3209) (9, 16, 16.3209) (9, 16, 10.3209)
fillet "Fillet4" radius 2 2 edges at (0, 17, 1) (40, 17, 1)

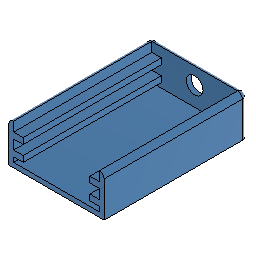
design "Base Staion Enclosure V2"
Autodesk Fusion 360 part; units mm, degrees
sketch "Sketch1" plane through (0, 0, 0) normal (0, 0, 1) x (1, 0, 0)
  line L0 (0, 0) -> (40, 0)
  line L1 (40, 0) -> (40, 60)
  line L2 (40, 60) -> (0, 60)
  line L3 (0, 60) -> (0, 0)
  line L4 (0, 60) -> (2, 60)
  line L5 (2, 60) -> (2, 58)
  line L6 (40, 0) -> (38, 0)
  line L7 (38, 0) -> (38, 2)
  line L8 (2, 58) -> (38, 58)
  line L9 (38, 58) -> (38, 2)
  line L10 (38, 2) -> (2, 2)
  line L11 (2, 2) -> (2, 58)
  line L12 (0, 60) -> (-10, 60)
  line L13 (-10, 60) -> (-10, 45)
  line L14 (-10, 45) -> (0, 45)
  line L15 (20, 60) -> (20, 87)
  line L16 (50, 60) -> (50, 45)
  line L17 (50, 45) -> (40, 45)
  line L18 (40, 60) -> (50, 60)
  line L19 (-10, 60) -> (-7, 60)
  line L20 (0, 60) -> (-2, 60)
  line L21 (-2, 60) -> (-2, 45)
  line L22 (-10, 45) -> (-7, 45)
  line L23 (-7, 45) -> (-7, 48)
  line L24 (-7, 48) -> (-2, 48)
  line L25 (-7, 60) -> (-7, 57)
  line L26 (-7, 57) -> (-2, 57)
  line L27 (-7, 57) -> (-7, 48)
  line L28 (-2, 57) -> (0, 57)
  line L29 (-2, 48) -> (0, 48)
  dimension "d1" = 40
  dimension "d2" = 60
  dimension "d3" = 2
  dimension "d4" = 2
  dimension "d5" = 2
  dimension "d6" = 2
  dimension "d40" = 10
  dimension "d41" = 15
  dimension "d60" = 3
  dimension "d61" = 2
  dimension "d62" = 3
  dimension "d63" = 3
  dimension "d64" = 3
  constraint horizontal L0
  constraint vertical L1
  constraint horizontal L2
  constraint vertical L3
  constraint coincident L0.start L3.end
  constraint perpendicular L3 L4
  constraint perpendicular L2 L5
  constraint perpendicular L1 L6
  constraint perpendicular L6 L7
  constraint horizontal L8
  constraint vertical L9
  constraint horizontal L10
  constraint vertical L11
  constraint perpendicular L3 L12
  constraint perpendicular L2 L13
  constraint coincident L3 L14.end
  constraint perpendicular L3 L14
  constraint midpoint L2 L15.start
  constraint perpendicular L2 L15
  constraint symmetric L2.end L15 L1.end
  constraint symmetric L12.end L15 L16.start
  constraint symmetric L13.end L15 L16.end
  constraint symmetric L14.end L15 L17.end
  constraint coincident L12 L19.end
  constraint perpendicular L3 L20
  constraint coincident L14 L21.end
  constraint perpendicular L14 L21
  constraint perpendicular L13 L22
  constraint perpendicular L22 L23
  constraint coincident L21 L24.end
  constraint perpendicular L21 L24
  constraint perpendicular L19 L25
  constraint coincident L21 L26.end
  constraint perpendicular L21 L26
  constraint coincident L3 L28.end
  constraint perpendicular L3 L28
  constraint coincident L3 L29.end
  constraint perpendicular L3 L29
  measures "d1" distance of L0.start L0.end
  measures "d2" distance of L0.start L2.end
  measures "d3" distance of L2.end L4.end
  measures "d4" distance of L4.end L5.end
  measures "d5" distance of L0.end L6.end
  measures "d6" distance of L6.end L7.end
  measures "d40" distance of L2.end L12.end
  measures "d41" distance of L12.end L13.end
  measures "d60" distance of L12.end L19.end
  measures "d61" distance of L2.end L20.end
  measures "d62" distance of L13.end L22.end
  measures "d63" distance of L22.end L23.end
  measures "d64" distance of L19.end L25.end
extrude "Extrude1" add sketch "Sketch1" along normal blind 2 contours L8 L9 L10 L11
extrude "Extrude2" add sketch "Sketch1" along normal blind 25 contours L0 L2 L3 L4 L5 L7 L10 L11 | L0 L1 L2 L5 L6 L7 L8 L9
sketch "Sketch6" plane through (0, 0, 25) normal (0, 0, 1) x (-1, 0, 0)
  line L0 (-38, -2) -> (-2, -2)
  line L1 (-2, -2) -> (-2, -58)
  line L2 (-2, -58) -> (-38, -58)
  line L3 (-38, -58) -> (-38, -2)
  line L4 (-40, -60) -> (0, -60)
  line L5 (0, -60) -> (0, 0)
  line L6 (0, 0) -> (-40, 0)
  line L7 (-40, 0) -> (-40, -60)
  line L8 (-38, -2) -> (-38, 0)
  line L9 (-2, -2) -> (-2, 0)
  constraint coincident L0.start L3.end
  constraint coincident L6 L8.end
  constraint perpendicular L6 L8
  constraint coincident L0.end L1.start
  constraint coincident L6 L9.end
  constraint perpendicular L0 L9
extrude "Extrude10" cut sketch "Sketch6" against normal blind 23 contours L0 L6 L8 L9
sketch "Sketch7" plane through (0, 0, 0) normal (0, -1, 0) x (1, 0, 0)
  line L0 (2, 2) -> (2, 25)
  line L1 (2, 25) -> (0, 25)
  line L2 (0, 25) -> (0, 0)
  line L3 (0, 0) -> (40, 0)
  line L4 (40, 0) -> (40, 25)
  line L5 (40, 25) -> (38, 25)
  line L6 (38, 25) -> (38, 2)
  line L7 (38, 2) -> (2, 2)
  line L8 (2, 2) -> (2, 4)
  line L9 (2, 4) -> (6, 4)
  line L10 (6, 4) -> (6, 6.5)
  line L11 (6, 6.5) -> (2, 6.5)
  line L12 (2, 25) -> (2, 13)
  line L13 (2, 13) -> (6, 13)
  line L14 (6, 13) -> (6, 10.5)
  line L15 (6, 10.5) -> (2, 10.5)
  line L16 (20, 0) -> (20, -5)
  line L17 (38, 4) -> (34, 4)
  line L18 (34, 4) -> (34, 6.5)
  line L19 (34, 6.5) -> (38, 6.5)
  line L20 (34, 10.5) -> (38, 10.5)
  line L21 (34, 13) -> (34, 10.5)
  line L22 (38, 13) -> (34, 13)
  dimension "d75" = 2
  dimension "d76" = 4
  dimension "d77" = 2.5
  dimension "d78" = 12
  dimension "d79" = 4
  dimension "d80" = 2.5
  constraint coincident L0.start L7.end
  constraint perpendicular L7 L8
  constraint perpendicular L8 L9
  constraint perpendicular L9 L10
  constraint coincident L0 L11.end
  constraint perpendicular L0 L11
  constraint coincident L0.end L1.start
  constraint coincident L0 L12.end
  constraint perpendicular L12 L13
  constraint perpendicular L13 L14
  constraint coincident L0 L15.end
  constraint perpendicular L0 L15
  constraint midpoint L3 L16.start
  constraint perpendicular L3 L16
  constraint symmetric L8.end L16 L17.start
  constraint symmetric L9.end L16 L17.end
  constraint symmetric L10.end L16 L18.end
  constraint symmetric L11.end L16 L19.end
  constraint symmetric L12.end L16 L22.start
  constraint symmetric L13.end L16 L21.start
  constraint symmetric L14.end L16 L20.start
  constraint symmetric L15.end L16 L20.end
  measures "d75" distance of L0.start L8.end
  measures "d76" distance of L8.end L9.end
  measures "d77" distance of L9.end L10.end
  measures "d78" distance of L0.end L12.end
  measures "d79" distance of L12.end L13.end
  measures "d80" distance of L13.end L14.end
extrude "Extrude11" add sketch "Sketch7" against normal blind 58 contours L0 L9 L10 L11 | L6 L17 L18 L19 | L0 L13 L14 L15 | L6 L20 L21 L22
sketch "Sketch8" plane through (0, 0, 0) normal (0, -1, 0) x (1, 0, 0)
  line L0 (0, 25) -> (0, 0)
  line L1 (0, 0) -> (40, 0)
  line L2 (40, 0) -> (40, 25)
  line L3 (38, 25) -> (38, 13)
  line L4 (38, 13) -> (34, 13)
  line L5 (34, 13) -> (34, 10.5)
  line L6 (34, 10.5) -> (38, 10.5)
  line L7 (38, 10.5) -> (38, 6.5)
  line L8 (38, 6.5) -> (34, 6.5)
  line L9 (34, 6.5) -> (34, 4)
  line L10 (34, 4) -> (38, 4)
  line L11 (38, 4) -> (38, 2)
  line L12 (38, 2) -> (2, 2)
  line L13 (2, 2) -> (2, 4)
  line L14 (2, 4) -> (6, 4)
  line L15 (6, 4) -> (6, 6.5)
  line L16 (6, 6.5) -> (2, 6.5)
  line L17 (2, 6.5) -> (2, 10.5)
  line L18 (2, 10.5) -> (6, 10.5)
  line L19 (6, 10.5) -> (6, 13)
  line L20 (6, 13) -> (2, 13)
  line L21 (2, 13) -> (2, 25)
  line L22 (0, 0) -> (0, 17)
  line L23 (0, 17) -> (40, 17)
  line L24 (0, 17) -> (49.5328, 17)
  line L25 (49.5328, 17) -> (49.5328, 30.8118)
  line L26 (49.5328, 30.8118) -> (0, 30.8118)
  line L27 (0, 30.8118) -> (0, 17)
  line L28 (2, 25) -> (0, 25)
  line L29 (40, 25) -> (38, 25)
  dimension "d87" = 17
  constraint coincident L0.end L1.start
  constraint perpendicular L1 L22
  constraint coincident L2 L23.end
  constraint perpendicular L2 L23
  constraint horizontal L24
  constraint vertical L25
  constraint horizontal L26
  constraint vertical L27
  measures "d87" distance of L0.end L22.end
extrude "Extrude13" cut sketch "Sketch8" against normal blind 78 contours L0 L21 L23 L24 L27 L28 | L2 L3 L21 L23 L24 L25 L26 L27 L28 L29 | L2 L3 L23 L24 L29
fillet "Fillet13" radius 2 2 edges at (0, 30, 17) (40, 30, 17)
sketch "Sketch9" plane through (0, 60, 0) normal (0, 1, 0) x (-1, 0, 0)
  arc A0 (-38, 17) -> (-40, 15) centre (-38, 15) ccw
  line L0 (-40, 15) -> (-40, 0)
  line L1 (-40, 0) -> (0, 0)
  line L2 (0, 0) -> (0, 15)
  arc A1 (0, 15) -> (-2, 17) centre (-2, 15) ccw
  line L3 (-2, 17) -> (-38, 17)
  line L4 (-20, 0) -> (-20, 10)
  circle A2 centre (-20, 10) radius 3.5
  dimension "d92" = 10
  dimension "d93" = 7
  constraint midpoint L1 L4.start
  constraint perpendicular L1 L4
  constraint coincident L4.end A2.centre
  measures "d92" distance of L4.start L4.end
  measures "d93" diameter of A2
extrude "Extrude14" cut sketch "Sketch9" against normal blind 2 contours A2
fillet "Fillet14" radius 2 5 edges at (40, 60, 7.5) (39.4142, 60, 16.4142) (20, 60, 17) (0.5858, 60, 16.4142) (0, 60, 7.5)
